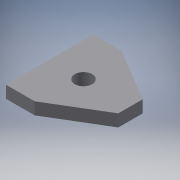
# Autodesk Inventor part: 30_Cube_Z_Focus_Drylin_NEMA_slide_part1
Saved by Autodesk Inventor 2019.4 (Build 234330000, 330)
## iProperties
Created: 2021-05-05
Part Number: 30_Cube_Z_Focus_Drylin_NEMA_slide_part1
Material: Generic
Document SubType Name: Modeling
Designer: diederichbenedict
Density: 1 g/cm^3
Appearance: Default
Author: diederichbenedict
Autodesk Inventor part; units mm, degrees
ref_plane "YZ Plane" through (0, 0, 0) normal (1, 0, 0) x (0, 1, 0)
ref_plane "XZ Plane" through (0, 0, 0) normal (0, 1, 0) x (-1, 0, 0)
ref_plane "XY Plane" through (0, 0, 0) normal (0, 0, 1) x (1, 0, 0)
sketch "Sketch1" plane through (0, 0, 0) normal (0, 1, 0) x (-1, 0, 0)
  line L0 (-13.5, -12.4952) -> (9.75, -12.4952)
  line L1 (9.75, -12.4952) -> (9.75, 12.4952)
  line L2 (9.75, 12.4952) -> (-13.5, 12.4952)
  line L3 (-13.5, 12.4952) -> (-13.5, -12.4952)
  circle A0 centre (-7.5, 0) radius 4
  circle A1 centre (3.75, -6.4952) radius 4
  circle A2 centre (3.75, 6.4952) radius 4
  line L4 (-2.75, -1.5877) -> (-2.75, 1.5877)
  line L5 (-2.75, 1.5877) -> (0, 3.1754)
  line L6 (0, 3.1754) -> (2.75, 1.5877)
  line L7 (2.75, 1.5877) -> (2.75, -1.5877)
  line L8 (2.75, -1.5877) -> (0, -3.1754)
  line L9 (0, -3.1754) -> (-2.75, -1.5877)
  circle A3 centre (0, 0) radius 7.5 construction
  dimension "d11" = 15
  dimension "d2" = 8
  dimension "d6" = 360
  dimension "d8" = 6
  dimension "d9" = 6
  dimension "d10" = 5.5
  dimension "d12" = 6
  dimension "d13" = 6
  constraints: 20 end point, 3 centre point, 3 parallel, 2 coincident, 1 horizontal, 1 horizontal alignment, 1 perpendicular, 22 other
  measures "d2" diameter of A0
  measures "d8" distance from line of A2.centre L1
  measures "d9" distance from line of L3 A0.centre
  measures "d10" distance between parallel lines of L4 L7
  measures "d12" distance from line of L2 A2.centre
  measures "d13" distance from line of L0 A1.centre
extrude "Extrusion1" add sketch "Sketch1" along normal blind 3 contours L3 L2 L1 L0 | L4 L5 L6 L7 L8 L9
sketch "Sketch2" plane through (0, 3, 0) normal (0, 1, 0) x (1, 0, 0)
  circle A0 centre (-3.75, -6.4952) radius 4 projected
  circle A1 centre (-3.75, 6.4952) radius 4 projected
  circle A2 centre (7.5, 0) radius 4 projected
  line L0 (13.5, 12.4952) -> (-9.75, 12.4952) projected
  line L1 (-9.75, 12.4952) -> (-9.75, -12.4952) projected
  line L2 (-9.75, -12.4952) -> (13.5, -12.4952) projected
  line L3 (13.5, -12.4952) -> (13.5, 12.4952) projected
  circle A3 centre (0, 0) radius 2.5
  dimension "d16" = 5
  constraints: 1 centre point, 1 coincident
  measures "d16" diameter of A3
extrude "Extrusion2" add sketch "Sketch2" along normal blind 0.5 contours A0 | A1 | A2 | L3 L2 L1 L0
sketch "Sketch3" plane through (0, 0, 0) normal (0, -1, 0) x (1, 0, 0)
  circle A0 centre (-3.75, 6.4952) radius 4 projected
  circle A1 centre (-3.75, -6.4952) radius 4 projected
  circle A2 centre (7.5, 0) radius 4 projected
  line L0 (13.5, -12.4952) -> (-9.75, -12.4952) projected
  line L1 (13.5, 12.4952) -> (13.5, -12.4952) projected
  line L2 (-9.75, 12.4952) -> (13.5, 12.4952) projected
  line L3 (-9.75, -12.4952) -> (-9.75, 12.4952) construction
  line L4 (-1.5, 12.4952) -> (13.5, 3.4952)
  line L5 (13.5, 12.4952) -> (13.5, -12.4952) projected
  line L6 (13.5, -3.4952) -> (-1.5, -12.4952)
  circle A3 centre (0, 0) radius 2.5 projected
  dimension "d19" = 9
  dimension "d20" = 9
  dimension "d21" = 15
  dimension "d22" = 15
  constraints: 4 end point, 4 point on line
  measures "d19" distance from line of L2 L4.end
  measures "d20" distance from line of L0 L6.start
  measures "d21" distance from line of L6.end L1
  measures "d22" distance from line of L1 L4.start
extrude "Extrusion3" cut sketch "Sketch3" against normal through all contours L4 L2 L1 | L0 L6 L1 | A3
body "Solid1"
